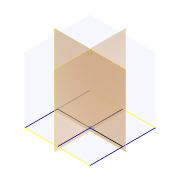
# Autodesk Inventor part: robot
Saved by Autodesk Inventor 2018 (Build 220112000, 112)
## iProperties
Created: 2019-01-20
Part Number: robot
Material: Generic
Document SubType Name: Modeling
Designer: ball
Density: 1 g/cm^3
Appearance: Default
Author: ball
Autodesk Inventor part; units mm, degrees
ref_plane "YZ Plane" through (0, 0, 0) normal (1, 0, 0) x (0, 1, 0)
ref_plane "XZ Plane" through (0, 0, 0) normal (0, 1, 0) x (-1, 0, 0)
ref_plane "XY Plane" through (0, 0, 0) normal (0, 0, 1) x (1, 0, 0)
sketch "Sketch1" plane through (0, 0, 0) normal (0, 1, 0) x (-1, 0, 0)
  line L0 (228.6, 228.6) -> (-228.6, 228.6)
  line L1 (-228.6, 228.6) -> (-228.6, -228.6)
  line L2 (-228.6, -228.6) -> (228.6, -228.6)
  line L3 (228.6, -228.6) -> (228.6, 228.6)
  point P0 (0, 0)
  dimension "d0" = 457.2
  dimension "d1" = 457.2
  constraints: 8 end point, 2 parallel, 1 horizontal, 1 perpendicular
  measures "d0" distance of L2.end L1.end
  measures "d1" distance of L1.end L0.end
extrude "Extrusion1" add sketch "Sketch1" along normal blind 457.2
sketch "Sketch3" plane through (0, 0, 0) normal (0, -1, 0) x (1, 0, 0)
  line L0 (-228.6, 228.6) -> (228.6, 228.6) projected
  line L1 (0, 228.6) -> (0, -228.6)
  line L2 (228.6, -228.6) -> (-228.6, -228.6) projected
  line L3 (228.6, 0) -> (-228.6, 0)
  line L4 (228.6, 228.6) -> (228.6, -228.6)
  line L5 (-228.6, 228.6) -> (-228.6, -228.6)
  point P0 (0, 0)
  point P1 (0, 0)
  constraints: 8 end point, 2 midpoint, 1 coincident, 1 horizontal, 1 parallel, 1 perpendicular
ref_plane "Work Plane1" through (-228.6, 0, 0) normal (0, 0, 1) x (1, 0, 0)
ref_plane "Work Plane2" through (0, 0, 228.6) normal (1, 0, 0) x (0, 0, -1)
sketch "Sketch4" plane through (0, 457.2, 0) normal (0, 1, 0) x (1, 0, 0)
  point P0 (0, 0)
  point P1 (0, 0)
  constraints: 1 coincident
sketch "Sketch5" plane through (0, 0, 0) normal (0, -1, 0) x (1, 0, 0)
  circle A0 centre (0, 0) radius 3.175
  dimension "d4" = 6.35
  constraints: 1 centre point, 1 coincident
  measures "d4" diameter of A0
body "Solid1"
